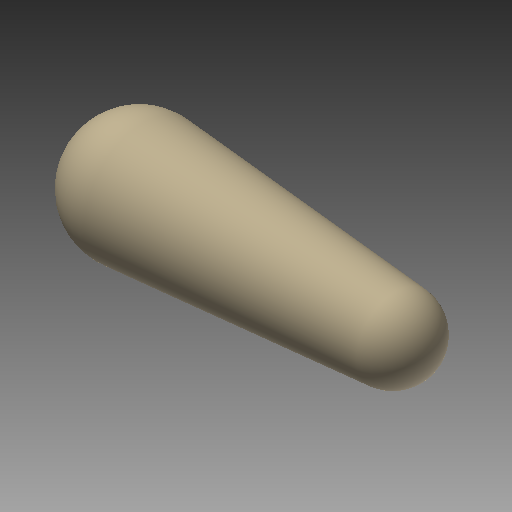
# Autodesk Inventor part: 3D HUMAN
Saved by Autodesk Inventor 2019 (Build 230136000, 136)
## iProperties
Category: PART
Company: Cross Bros.
Shininess: 64.0
Length Units: 11272
Angle Units: 11279
Time Units: 11290
Mass Units: 11286
Length Display Precision: 3
Angle Display Precision: 2
Compacted: True
Part Number: 3D HUMAN
Document SubType Name: Modeling
Created: 2003-03-23
Designer: M.F.
Catalog Web Link: www.apollocanard.com
Density: 1 g/cm^3
Material: Generic
Appearance: Beige
Density: 0.0
Volumn: 0.0
Area: 0.0
PropertySet Name: Model Information
Control State: 0
Master: False
Checked Out: False
Title: iMan
Author: M.F.
Autodesk Inventor part; units mm, degrees
ref_plane "YZ Plane" through (0, 0, 0) normal (1, 0, 0) x (0, 1, 0)
ref_plane "XZ Plane" through (0, 0, 0) normal (0, 1, 0) x (-1, 0, 0)
ref_plane "XY Plane" through (0, 0, 0) normal (0, 0, 1) x (1, 0, 0)
sketch "Sketch1" plane through (0, 0, 0) normal (0, 0, 1) x (1, 0, 0)
  circle A0 centre (0, 0) radius 92.329
  circle A1 centre (0, -391.16) radius 61.468
  line L0 (0, 92.329) -> (0, -452.628)
  line L1 (92.0412, -7.2844) -> (61.2764, -396.0096)
  dimension "d16" = 391.16
  dimension "d17" = 184.658
  dimension "d18" = 122.936
  constraints: 4 end point, 4 point on circle, 2 centre point, 2 tangent, 1 coincident, 1 point on line, 1 vertical, 1 vertical alignment
  measures "d16" distance of A1.centre A0.centre
  measures "d17" diameter of A0
  measures "d18" diameter of A1
revolve "Revolution1" add sketch "Sketch1" angle 360 about axis through (0, 92.329, 0) along (0, -1, 0) picked at (24.5341, 22.9459) picked at (20.0187, -411.9129) contours A0 L0 | L1 A1 L0 A0 | A1 L0
equation "\"d16\" = PELVIS_TO_KNEE"
equation "\"d17\" = LEG_TOP_THK"
equation "\"d18\" = KNEE_THK"
equation "\"PELVIS_TO_KNEE\" = 391.16"
equation "\"LEG_TOP_THK\" = 184.658"
equation "\"KNEE_THK\" = 122.936"
body "Solid1"
